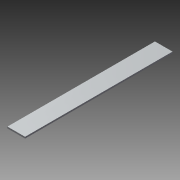
# Autodesk Inventor part: small side
Saved by Autodesk Inventor 2015 (Build 190159000, 159)
## iProperties
Created: 2015-01-31
Part Number: small side
Material: Generic
Document SubType Name: Modeling
Designer: Joseph
Density: 1 g/cm^3
Appearance: Default
Author: Joseph
Autodesk Inventor part; units mm, degrees
ref_plane "YZ Plane" through (0, 0, 0) normal (1, 0, 0) x (0, 1, 0)
ref_plane "XZ Plane" through (0, 0, 0) normal (0, 1, 0) x (-1, 0, 0)
ref_plane "XY Plane" through (0, 0, 0) normal (0, 0, 1) x (1, 0, 0)
sketch "Sketch1" plane through (0, 0, 0) normal (0, 0, 1) x (1, 0, 0)
  line L0 (0, 20) -> (25.8492, 20) projected
  line L1 (25.8492, 0) -> (25.8492, 20) projected
  line L2 (-45.8684, 0) -> (-45.8684, 20) projected
  line L3 (-20.0191, -580) -> (-45.8684, -580) projected
  line L4 (-45.8684, -580) -> (25.8492, -580)
  line L5 (25.8492, -580) -> (25.8492, 20)
  line L6 (25.8492, 20) -> (-45.8684, 20)
  line L7 (-45.8684, 20) -> (-45.8684, -580)
  point P0 (0, 0)
  constraints: 8 end point, 2 parallel, 1 horizontal, 1 perpendicular
extrude "Extrusion1" add sketch "Sketch1" along normal blind 6.35
body "Solid1"
